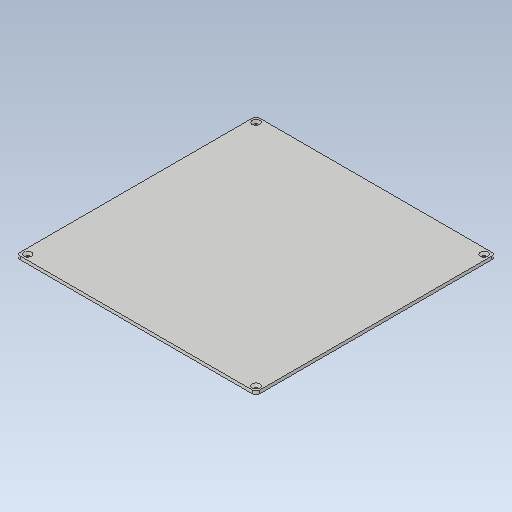
# Autodesk Inventor part: 20_stół
Saved by Autodesk Inventor 2020.2 (Build 242310000, 310)
## iProperties
Created: 2017-10-23
Part Number: 20_stół
Material: Ogólny
Document SubType Name: Modeling
Designer: Haras
Density: 1 g/cm^3
Appearance: Domyślna
Author: Haras
Autodesk Inventor part; units mm, degrees
ref_plane "YZ Plane" through (0, 0, 0) normal (1, 0, 0) x (0, 1, 0)
ref_plane "XZ Plane" through (0, 0, 0) normal (0, 1, 0) x (-1, 0, 0)
ref_plane "XY Plane" through (0, 0, 0) normal (0, 0, 1) x (1, 0, 0)
sketch "Szkic1" plane through (0, 0, 0) normal (0, 1, 0) x (-1, 0, 0)
  line L0 (110, 110) -> (-110, 110)
  line L1 (-110, 110) -> (-110, -110)
  line L2 (-110, -110) -> (110, -110)
  line L3 (110, -110) -> (110, 110)
  line L4 (110, 0) -> (-110, 0) construction
  line L5 (0, 110) -> (0, -110) construction
  point P0 (0, 0)
  dimension "d0" = 220
  dimension "d1" = 220
  constraints: 12 end point, 6 midpoint, 2 parallel, 1 horizontal, 1 perpendicular
  measures "d0" distance of L2.end L0.start
  measures "d1" distance of L1.end L2.end
extrude "Wyciągnięcie proste1" add sketch "Szkic1" along normal blind 3
sketch "Szkic2" plane through (0, 3, 0) normal (0, 1, 0) x (1, 0, 0)
  line L0 (-110, 110) -> (-110, -110) projected
  line L1 (-110, -110) -> (110, -110) projected
  line L2 (110, -110) -> (110, 110) projected
  line L3 (110, 110) -> (-110, 110) projected
  point P0 (0, 0)
  point P1 (-105, -105)
  point P2 (-105, 105)
  point P3 (105, 105)
  point P4 (105, -105)
  dimension "d4" = 5
  dimension "d5" = 5
  dimension "d6" = 5
  dimension "d7" = 5
  constraints: 2 horizontal alignment, 2 vertical alignment
  measures "d4" distance from line of L0 point (-105, -105)
  measures "d5" distance from line of L1 point (-105, -105)
  measures "d6" distance from line of L2 point (105, 105)
  measures "d7" distance from line of L3 point (105, 105)
hole "Otwór1" at (-105, 3, 105) at (-105, 3, -105) at (105, 3, -105) at (105, 3, 105) direction (0, -1, 0) diameter 3 end through all
fillet "Zaokrąglenie1" radius 3 4 edges at (-110, 1.5, 110) (110, 1.5, 110) (110, 1.5, -110) (-110, 1.5, -110)
chamfer "Faza1" distance 2 angle 45 4 edges at (105, 3, -106.5) (-105, 3, -106.5) (105, 3, 103.5) (-105, 3, 103.5)
